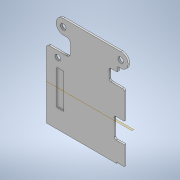
# Autodesk Inventor part: kommutation_board
Saved by Autodesk Inventor 2022 (Build 260153000, 153)
## iProperties
Created: 2024-12-13
Part Number: kommutation_board
Material: Типовые
Document SubType Name: Modeling
Designer: Andrey
Density: 1 g/cm^3
Appearance: По умолчанию
Author: Andrey
Autodesk Inventor part; units mm, degrees
ref_plane "YZ Plane" through (0, 0, 0) normal (1, 0, 0) x (0, 1, 0)
ref_plane "XZ Plane" through (0, 0, 0) normal (0, 1, 0) x (-1, 0, 0)
ref_plane "XY Plane" through (0, 0, 0) normal (0, 0, 1) x (1, 0, 0)
sketch "Эскиз1" plane through (0, 0, 0) normal (0, 0, 1) x (1, 0, 0)
  line L0 (-7.7719, -54) -> (-12.7719, -54) projected
  line L1 (-12.7719, -54) -> (-12.7719, -40.5) projected
  line L2 (-12.7719, -40.5) -> (-7.7719, -40.5) projected
  line L3 (-7.7719, -40.5) -> (-7.7719, -54) projected
  circle A0 centre (-17.7467, 10.9) radius 1.6 projected
  circle A1 centre (-17.7467, -40.1) radius 1.6 projected
  arc A2 (20.7533, -26.4) -> (20.2533, -25.9) centre (20.2533, -26.4) ccw projected
  line L4 (20.2533, -25.9) -> (-21.1, -25.9) projected
  arc A3 (-23.1, -23.9) -> (-21.1, -25.9) centre (-21.1, -23.9) ccw projected
  line L5 (-23.1, -23.9) -> (-23.1, -2.3) projected
  arc A4 (-21.1, -0.3) -> (-23.1, -2.3) centre (-21.1, -2.3) ccw projected
  line L6 (-21.1, -0.3) -> (-13.1, -0.3) projected
  arc A5 (-13.1, -0.3) -> (-11.1, 1.7) centre (-13.1, 1.7) ccw projected
  line L7 (-11.1, 1.7) -> (-11.1, 15.1) projected
  arc A6 (-11.1, 15.1) -> (-13.1, 17.1) centre (-13.1, 15.1) ccw projected
  line L8 (-13.1, 17.1) -> (-15.05, 17.1) projected
  arc A7 (-18.0974, 25.0287) -> (-15.05, 17.1) centre (-15.05, 21.65) ccw projected
  arc A8 (-18.0974, 25.0287) -> (-18.4323, 25.9) centre (-18.4323, 25.4) ccw projected
  line L9 (-25.3018, 25.9) -> (-18.4323, 25.9) projected
  line L10 (-25.3018, 25.9) -> (-25.3018, 22.9) projected
  line L11 (-26.6467, 22.9) -> (-25.3018, 22.9) projected
  line L12 (-26.6467, -42.7) -> (-26.6467, 22.9) projected
  line L13 (-26.6467, -42.7) -> (-18.7719, -42.7) projected
  line L14 (-18.7719, -42.7) -> (-18.7719, -54.2) projected
  line L15 (-18.7719, -54.2) -> (-25.3018, -54.2) projected
  line L16 (-25.3018, -54.2) -> (-25.3018, -55.1) projected
  line L17 (31.7533, -55.1) -> (-25.3018, -55.1) projected
  line L18 (31.7533, -55.1) -> (31.7533, -46.6) projected
  line L19 (31.7533, -46.6) -> (17.9318, -46.6) projected
  spline S0 degree 3 poles (17.3769, -46.1) (17.3769, -46.1597) (17.3919, -46.2298) (17.441, -46.342) (17.485, -46.4032) (17.5795, -46.4922) (17.6478, -46.5345) (17.7766, -46.5847) (17.8606, -46.6) (17.9318, -46.6) knots 0 0 0 0 0.017914 0.017914 0.036753 0.036753 0.056849 0.056849 0.078208 0.078208 0.078208 0.078208 projected
  line L20 (17.3769, -46.1) -> (17.3769, -44.1) projected
  spline S1 degree 3 poles (16.8292, -43.6) (16.8984, -43.6) (16.9801, -43.6153) (17.1065, -43.6649) (17.1743, -43.7071) (17.2685, -43.796) (17.3126, -43.8574) (17.3619, -43.9699) (17.3769, -44.0401) (17.3769, -44.1) knots 0.386783 0.386783 0.386783 0.386783 0.407551 0.407551 0.427519 0.427519 0.446405 0.446405 0.464367 0.464367 0.464367 0.464367 projected
  line L21 (16.8292, -43.6) -> (14.9, -43.6) projected
  line L22 (14.9, -43.6) -> (14.9, -36.8) projected
  line L23 (14.9, -36.8) -> (31.7533, -36.8) projected
  line L24 (31.7533, -36.8) -> (31.7533, -32.1) projected
  line L25 (31.7533, -32.1) -> (20.7533, -32.1) projected
  line L26 (20.7533, -32.1) -> (20.7533, -26.4) projected
  arc A9 (21.8974, 18.2713) -> (22.2323, 17.4) centre (22.2323, 17.9) ccw projected
  line L27 (22.2323, 17.4) -> (31.7533, 17.4) projected
  line L28 (31.7533, 17.4) -> (31.7533, 25.9) projected
  line L29 (22.2323, 25.9) -> (31.7533, 25.9) projected
  arc A10 (22.2323, 25.9) -> (21.8974, 25.0287) centre (22.2323, 25.4) ccw projected
  arc A11 (21.8974, 18.2713) -> (21.8974, 25.0287) centre (18.85, 21.65) ccw projected
  line L30 (21.5533, 2.9) -> (31.7533, 2.9) projected
  line L31 (31.7533, 2.9) -> (31.7533, 7.6) projected
  line L32 (31.7533, 7.6) -> (21.5533, 7.6) projected
  line L33 (7.4642, -8.6) -> (7.4642, -4.1) projected
  line L34 (20.7533, -8.6) -> (7.4642, -8.6) projected
  line L35 (20.7533, 2.9) -> (20.7533, -8.6) projected
  line L36 (21.5533, 2.9) -> (20.7533, 2.9) projected
  line L37 (14.9, 7.6) -> (21.5533, 7.6) projected
  line L38 (14.9, -1.1) -> (14.9, 7.6) projected
  arc A12 (11.9, -4.1) -> (14.9, -1.1) centre (11.9, -1.1) ccw projected
  line L39 (7.4642, -4.1) -> (11.9, -4.1) projected
  line L40 (7.4642, -4.1) -> (11.9, -4.1) projected
  circle A13 centre (-15.05, 21.65) radius 1.5 projected
  line L41 (-18.4323, 25.9) -> (-11.1, 25.9) projected
  arc A14 (-18.0974, 25.0287) -> (-18.4323, 25.9) centre (-18.4323, 25.4) ccw projected
  arc A15 (-18.0974, 25.0287) -> (-15.05, 17.1) centre (-15.05, 21.65) ccw projected
  line L42 (-13.1, 17.1) -> (-15.05, 17.1) projected
  arc A16 (-11.1, 15.1) -> (-13.1, 17.1) centre (-13.1, 15.1) ccw projected
  line L43 (-11.1, 25.9) -> (-11.1, 15.1) projected
  line L44 (14.9, 25.9) -> (22.2323, 25.9) projected
  line L45 (14.9, 14.4) -> (14.9, 25.9) projected
  line L46 (16.4121, 14.4) -> (14.9, 14.4) projected
  spline S2 degree 3 poles (16.9309, 14.9) (16.9309, 14.839) (16.9162, 14.7674) (16.8681, 14.654) (16.8258, 14.5925) (16.7358, 14.5046) (16.6718, 14.463) (16.5529, 14.4148) (16.4768, 14.4) (16.4121, 14.4) knots 0.150725 0.150725 0.150725 0.150725 0.169014 0.169014 0.187674 0.187674 0.206759 0.206759 0.226155 0.226155 0.226155 0.226155 projected
  line L47 (16.9309, 16.9) -> (16.9309, 14.9) projected
  spline S3 degree 3 poles (17.4522, 17.4) (17.3868, 17.4) (17.3098, 17.3852) (17.1901, 17.3368) (17.1259, 17.2952) (17.0358, 17.2072) (16.9935, 17.1458) (16.9455, 17.0325) (16.9309, 16.9609) (16.9309, 16.9) knots -0.075652 -0.075652 -0.075652 -0.075652 -0.056047 -0.056047 -0.036914 -0.036914 -0.018271 -0.018271 0 0 0 0 projected
  line L48 (22.2323, 17.4) -> (17.4522, 17.4) projected
  arc A17 (21.8974, 18.2713) -> (22.2323, 17.4) centre (22.2323, 17.9) ccw projected
  arc A18 (21.8974, 18.2713) -> (21.8974, 25.0287) centre (18.85, 21.65) ccw projected
  arc A19 (22.2323, 25.9) -> (21.8974, 25.0287) centre (22.2323, 25.4) ccw projected
  circle A20 centre (18.85, 21.65) radius 1.5 projected
  circle A21 centre (18.85, 21.65) radius 4.25
  circle A22 centre (-15.05, 21.65) radius 4.25
  line L49 (18.85, 25.9) -> (-15.05, 25.9)
  circle A23 centre (18.85, 21.65) radius 1.6
  circle A24 centre (-15.05, 21.65) radius 1.6
  line L50 (14.9, 7.6) -> (12.9, 7.6)
  line L51 (11.9, 8.6) -> (11.9, 13.4)
  line L52 (12.9, 14.4) -> (14.9, 14.4)
  line L53 (14.9, 14.4) -> (14.9, 7.6)
  line L54 (20.7533, -25.6) -> (-21.1, -25.6)
  arc A25 (-22.8, -23.9) -> (-21.1, -25.6) centre (-21.1, -23.9) ccw
  line L55 (-22.8, -23.9) -> (-22.8, -2.3)
  line L56 (-21.1, -0.6) -> (-13.1, -0.6)
  arc A26 (-13.1, -0.6) -> (-10.8, 1.7) centre (-13.1, 1.7) ccw
  arc A27 (-21.1, -0.6) -> (-22.8, -2.3) centre (-21.1, -2.3) ccw
  line L57 (-10.8, 1.7) -> (-10.8, 15.1)
  arc A28 (-10.8, 15.1) -> (-13.1, 17.4) centre (-13.1, 15.1) ccw
  line L58 (-13.1, 17.4) -> (-15.05, 17.4)
  arc A29 (21.0533, 3.4) -> (21.5533, 2.9) centre (21.5533, 3.4) ccw projected
  arc A30 (21.5533, 7.6) -> (21.0533, 7.1) centre (21.5533, 7.1) ccw projected
  line L59 (21.0533, 7.1) -> (21.0533, 3.4) projected
  arc A31 (21.0533, 3.4) -> (21.5533, 2.9) centre (21.5533, 3.4) ccw projected
  line L60 (21.0533, 7.1) -> (21.0533, 3.4) projected
  arc A32 (21.5533, 7.6) -> (21.0533, 7.1) centre (21.5533, 7.1) ccw projected
  line L61 (20.7533, 2.9) -> (20.7533, 6.6)
  line L62 (19.7533, 7.6) -> (14.9, 7.6)
  arc A33 (20.7533, 6.6) -> (19.7533, 7.6) centre (19.7533, 6.6) ccw
  arc A34 (11.9, 8.6) -> (12.9, 7.6) centre (12.9, 8.6) ccw
  arc A35 (12.9, 14.4) -> (11.9, 13.4) centre (12.9, 13.4) ccw
  line L63 (20.7533, -25.6) -> (20.7533, -20.6)
  line L64 (20.7533, -20.6) -> (15.9, -20.6)
  line L65 (20.7533, -8.6) -> (7.4642, -8.6) projected
  line L66 (20.7533, 2.9) -> (20.7533, -8.6) projected
  line L67 (21.5533, 2.9) -> (20.7533, 2.9) projected
  arc A36 (21.0533, 3.4) -> (21.5533, 2.9) centre (21.5533, 3.4) ccw projected
  line L68 (21.0533, 7.1) -> (21.0533, 3.4) projected
  arc A37 (21.5533, 7.6) -> (21.0533, 7.1) centre (21.5533, 7.1) ccw projected
  line L69 (14.9, 7.6) -> (21.5533, 7.6) projected
  line L70 (14.9, -1.1) -> (14.9, 7.6) projected
  arc A38 (11.9, -4.1) -> (14.9, -1.1) centre (11.9, -1.1) ccw projected
  line L71 (7.4642, -8.6) -> (7.4642, -4.1) projected
  arc A39 (14.9, -19.6) -> (15.9, -20.6) centre (15.9, -19.6) ccw projected
  line L72 (14.9, -19.6) -> (14.9, -9.6) projected
  arc A40 (15.9, -8.6) -> (14.9, -9.6) centre (15.9, -9.6) ccw projected
  line L73 (-7.7719, -54) -> (-12.7719, -54) projected
  line L74 (-12.7719, -54) -> (-12.7719, -40.5) projected
  line L75 (-12.7719, -40.5) -> (-7.7719, -40.5) projected
  line L76 (-7.7719, -40.5) -> (-7.7719, -54) projected
  circle A41 centre (-17.7467, 10.9) radius 1.6 projected
  circle A42 centre (-17.7467, -40.1) radius 1.6 projected
  arc A43 (20.7533, -26.4) -> (20.2533, -25.9) centre (20.2533, -26.4) ccw projected
  line L77 (20.2533, -25.9) -> (-21.1, -25.9) projected
  arc A44 (-23.1, -23.9) -> (-21.1, -25.9) centre (-21.1, -23.9) ccw projected
  line L78 (-23.1, -23.9) -> (-23.1, 4.7) projected
  arc A45 (-21.1, 6.7) -> (-23.1, 4.7) centre (-21.1, 4.7) ccw projected
  line L79 (-21.1, 6.7) -> (-13.1, 6.7) projected
  arc A46 (-13.1, 6.7) -> (-11.1, 8.7) centre (-13.1, 8.7) ccw projected
  line L80 (-11.1, 8.7) -> (-11.1, 15.1) projected
  arc A47 (-11.1, 15.1) -> (-13.1, 17.1) centre (-13.1, 15.1) ccw projected
  line L81 (-13.1, 17.1) -> (-15.05, 17.1) projected
  arc A48 (-18.0974, 25.0287) -> (-15.05, 17.1) centre (-15.05, 21.65) ccw projected
  arc A49 (-18.0974, 25.0287) -> (-18.4323, 25.9) centre (-18.4323, 25.4) ccw projected
  line L82 (-25.3018, 25.9) -> (-18.4323, 25.9) projected
  line L83 (-25.3018, 25.9) -> (-25.3018, 22.9) projected
  line L84 (-26.6467, 22.9) -> (-25.3018, 22.9) projected
  line L85 (-26.6467, -42.7) -> (-26.6467, 22.9) projected
  line L86 (-26.6467, -42.7) -> (-18.7719, -42.7) projected
  line L87 (-18.7719, -42.7) -> (-18.7719, -54.2) projected
  line L88 (-18.7719, -54.2) -> (-25.3018, -54.2) projected
  line L89 (-25.3018, -54.2) -> (-25.3018, -55.1) projected
  line L90 (31.7533, -55.1) -> (-25.3018, -55.1) projected
  line L91 (31.7533, -55.1) -> (31.7533, -46.6) projected
  line L92 (31.7533, -46.6) -> (17.9318, -46.6) projected
  spline S4 degree 3 poles (17.3769, -46.1) (17.3769, -46.1597) (17.3919, -46.2298) (17.441, -46.342) (17.485, -46.4032) (17.5795, -46.4922) (17.6478, -46.5345) (17.7766, -46.5847) (17.8606, -46.6) (17.9318, -46.6) knots 0 0 0 0 0.017914 0.017914 0.036753 0.036753 0.056849 0.056849 0.078208 0.078208 0.078208 0.078208 projected
  line L93 (17.3769, -46.1) -> (17.3769, -44.1) projected
  spline S5 degree 3 poles (16.8292, -43.6) (16.8984, -43.6) (16.9801, -43.6153) (17.1065, -43.6649) (17.1743, -43.7071) (17.2685, -43.796) (17.3126, -43.8574) (17.3619, -43.9699) (17.3769, -44.0401) (17.3769, -44.1) knots 0.386783 0.386783 0.386783 0.386783 0.407551 0.407551 0.427519 0.427519 0.446405 0.446405 0.464367 0.464367 0.464367 0.464367 projected
  line L94 (16.8292, -43.6) -> (14.9, -43.6) projected
  line L95 (14.9, -43.6) -> (14.9, -36.8) projected
  line L96 (14.9, -36.8) -> (31.7533, -36.8) projected
  line L97 (31.7533, -36.8) -> (31.7533, -32.1) projected
  line L98 (31.7533, -32.1) -> (20.7533, -32.1) projected
  line L99 (20.7533, -32.1) -> (20.7533, -26.4) projected
  line L100 (-10.8, 15.1) -> (-10.8, 8.7)
  arc A50 (-13.1, 6.4) -> (-10.8, 8.7) centre (-13.1, 8.7) ccw
  line L101 (-13.1, 6.4) -> (-21.1, 6.4)
  arc A51 (-21.1, 6.4) -> (-22.8, 4.7) centre (-21.1, 4.7) ccw
  line L102 (-22.8, 4.7) -> (-22.8, -23.9)
  line L103 (-7.7719, -54) -> (-12.7719, -54) projected
  line L104 (-12.7719, -54) -> (-12.7719, -40.5) projected
  line L105 (-12.7719, -40.5) -> (-7.7719, -40.5) projected
  line L106 (-7.7719, -40.5) -> (-7.7719, -54) projected
  circle A52 centre (-17.7467, 10.9) radius 1.6 projected
  circle A53 centre (-17.7467, -40.1) radius 1.6 projected
  arc A54 (20.7533, -29.4) -> (20.2533, -28.9) centre (20.2533, -29.4) ccw projected
  line L107 (20.2533, -28.9) -> (-21.1, -28.9) projected
  arc A55 (-23.1, -26.9) -> (-21.1, -28.9) centre (-21.1, -26.9) ccw projected
  line L108 (-23.1, -26.9) -> (-23.1, 4.7) projected
  arc A56 (-21.1, 6.7) -> (-23.1, 4.7) centre (-21.1, 4.7) ccw projected
  line L109 (-21.1, 6.7) -> (-13.1, 6.7) projected
  arc A57 (-13.1, 6.7) -> (-11.1, 8.7) centre (-13.1, 8.7) ccw projected
  line L110 (-11.1, 8.7) -> (-11.1, 15.1) projected
  arc A58 (-11.1, 15.1) -> (-13.1, 17.1) centre (-13.1, 15.1) ccw projected
  line L111 (-13.1, 17.1) -> (-15.05, 17.1) projected
  arc A59 (-18.0974, 25.0287) -> (-15.05, 17.1) centre (-15.05, 21.65) ccw projected
  arc A60 (-18.0974, 25.0287) -> (-18.4323, 25.9) centre (-18.4323, 25.4) ccw projected
  line L112 (-25.3018, 25.9) -> (-18.4323, 25.9) projected
  line L113 (-25.3018, 25.9) -> (-25.3018, 22.9) projected
  line L114 (-26.6467, 22.9) -> (-25.3018, 22.9) projected
  line L115 (-26.6467, -42.7) -> (-26.6467, 22.9) projected
  line L116 (-26.6467, -42.7) -> (-18.7719, -42.7) projected
  line L117 (-18.7719, -42.7) -> (-18.7719, -54.2) projected
  line L118 (-18.7719, -54.2) -> (-25.3018, -54.2) projected
  line L119 (-25.3018, -54.2) -> (-25.3018, -55.1) projected
  line L120 (31.7533, -55.1) -> (-25.3018, -55.1) projected
  line L121 (31.7533, -55.1) -> (31.7533, -46.6) projected
  line L122 (31.7533, -46.6) -> (17.9318, -46.6) projected
  spline S6 degree 3 poles (17.3769, -46.1) (17.3769, -46.1597) (17.3919, -46.2298) (17.441, -46.342) (17.485, -46.4032) (17.5795, -46.4922) (17.6478, -46.5345) (17.7766, -46.5847) (17.8606, -46.6) (17.9318, -46.6) knots 0 0 0 0 0.017914 0.017914 0.036753 0.036753 0.056849 0.056849 0.078208 0.078208 0.078208 0.078208 projected
  line L123 (17.3769, -46.1) -> (17.3769, -44.1) projected
  spline S7 degree 3 poles (16.8292, -43.6) (16.8984, -43.6) (16.9801, -43.6153) (17.1065, -43.6649) (17.1743, -43.7071) (17.2685, -43.796) (17.3126, -43.8574) (17.3619, -43.9699) (17.3769, -44.0401) (17.3769, -44.1) knots 0.386783 0.386783 0.386783 0.386783 0.407551 0.407551 0.427519 0.427519 0.446405 0.446405 0.464367 0.464367 0.464367 0.464367 projected
  line L124 (16.8292, -43.6) -> (14.9, -43.6) projected
  line L125 (14.9, -43.6) -> (14.9, -36.8) projected
  line L126 (14.9, -36.8) -> (31.7533, -36.8) projected
  line L127 (31.7533, -36.8) -> (31.7533, -32.1) projected
  line L128 (31.7533, -32.1) -> (20.7533, -32.1) projected
  line L129 (20.7533, -32.1) -> (20.7533, -29.4) projected
  line L130 (-22.8, 4.7) -> (-22.8, -26.9)
  arc A61 (-22.8, -26.9) -> (-21.1, -28.6) centre (-21.1, -26.9) ccw
  line L131 (-21.1, -28.6) -> (20.7533, -28.6)
  line L132 (21.0533, -29.4) -> (21.0533, -32.1)
  line L133 (20.7533, -28.6) -> (20.7533, -25.6)
  arc A62 (-23.3497, 8.2) -> (-25.3497, 6.2) centre (-23.3497, 6.2) ccw
  line L134 (-23.3497, 8.2) -> (-13.1, 8.2)
  arc A63 (-13.1, 8.2) -> (-11.1, 10.2) centre (-13.1, 10.2) ccw
  line L135 (-25.3497, 0.9) -> (-25.3497, 6.2)
  line L136 (-25.3499, -32.7) -> (-25.3499, 0.9)
  line L137 (16.4642, -32.7) -> (-25.3499, -32.7)
  line L138 (31.7533, -32.1) -> (16.4642, -32.1)
  line L139 (16.4642, -32.1) -> (16.4642, -32.7)
  line L140 (31.7533, -31.8) -> (16.1642, -31.8)
  line L141 (16.1642, -31.8) -> (16.1642, -32.4)
  line L142 (16.1642, -32.4) -> (-25.0499, -32.4)
  line L143 (-25.0499, -32.4) -> (-25.0499, 0.9)
  line L144 (-25.0497, 0.9) -> (-25.0497, 6.2)
  arc A64 (-23.3497, 7.9) -> (-25.0497, 6.2) centre (-23.3497, 6.2) ccw
  line L145 (-23.3497, 7.9) -> (-13.1, 7.9)
  arc A65 (-13.1, 7.9) -> (-10.8, 10.2) centre (-13.1, 10.2) ccw
  line L146 (-10.8, 10.2) -> (-10.8, 15.1)
  line L147 (20.7533, -28.6) -> (20.7533, -31.8)
  line L148 (20.7533, -28.6) -> (-21.1, -28.6)
  line L149 (-25.0499, -32.4) -> (16.1642, -32.4)
  line L150 (16.1642, -31.8) -> (16.1642, -32.4)
  line L151 (16.1642, -31.8) -> (20.7533, -31.8)
  line L152 (-25.0497, 6.2) -> (-25.0499, -32.4)
  line L153 (-10.8, 10.2) -> (-10.8, 1.7)
  point P0 (0, 0)
  point P1 (20.7533, 3.4)
  point P2 (20.7533, 7.1)
  point P3 (7.4642, -25.9)
  point P4 (-3.6642, -25.9)
  point P5 (11.9, 14.4)
  point P6 (20.7533, 7.6)
  point P7 (18.85, 17.4)
  point P8 (-22.8, -2.3)
  point P9 (-21.1, -25.6)
  point P10 (-11.1, 16.2358)
  point P11 (-22.8, -2.3)
  point P12 (20.7533, -26.4)
  point P13 (-11.1, 9.0642)
  point P14 (-22.8, -1.2464)
  point P15 (-22.8, -2.3)
  dimension "d0" = 3.2
  dimension "d1" = 3.2
  dimension "d2" = 3
  dimension "d3" = 0.3
  dimension "d4" = 0.3
  dimension "d5" = 0.3
  dimension "d6" = 0.3
  dimension "d7" = 0.3
  dimension "d8" = 0.3
  dimension "d9" = 0.3
  dimension "d10" = 0.3
  dimension "d11" = 0.3
  dimension "d12" = 1
  dimension "d13" = 1
  dimension "d20" = 0.3
  dimension "d22" = 0.3
  dimension "d26" = 0.3
  dimension "d27" = 0.3
  constraints: 82 end point, 28 point on circle, 16 centre point, 10 point on line, 10 tangent, 8 parallel, 6 horizontal, 5 perpendicular, 4 coincident, 4 vertical, 3 collinear, 1 equal radius, 32 other
  measures "d0" diameter of A23
  measures "d1" diameter of A24
  measures "d2" distance of point (11.9, 14.4) L52.end
  measures "d3" distance between parallel lines of L4 L54
  measures "d4" radial gap between concentric circles of A3 A25
  measures "d5" distance between parallel lines of L5 L55
  measures "d6" distance between parallel lines of L6 L56
  measures "d7" radial gap between concentric circles of A5 A26
  measures "d8" radial gap between concentric circles of A4 A27
  measures "d9" distance between parallel lines of L7 L57
  measures "d10" radial gap between concentric circles of A6 A28
  measures "d11" distance between parallel lines of L8 L58
  measures "d12" radius of A33
  measures "d13" radius of A34
  measures "d20" radial gap between concentric circles of A46 A50
  measures "d22" distance between parallel lines of L107 L131
  measures "d26" distance between parallel lines of L138 L140
  measures "d27" radial gap between concentric circles of A62 A64
extrude "Выдавливание1" add sketch "Эскиз1" along normal blind 1 contours L26 L131 A61 L130 A3 L4 A2 | A2 L4 A3 L130 A25 L54 L133 | L26 A54 L107 A55 L108 A3 L130 A61 L131 | L54 A25 L55 A27 L56 A26 L57 A28 L43 A22 L49 L45 A21 L52 A35 L51 A34 L50 L38 A12 L39 L33 L34 A40 L72 A39 L64 L63 | L26 L140 L141 L142 L143 L144 A64 L145 A65 L7 A46 L79 A45 L78 L5 L108 A55 L107 A54 | A3 L5 A4 L102 L55 L130 | L102 A4 L6 A5 L7 A50 L57 A26 L56 A27 | L78 A45 L79 A46 L7 A50 L101 A51 L102 A4 | L102 A51 L101 A50 L7 A5 L6 A4 | L34 L33 L39 A12 L38 L37 A33 L61 L35 | A50 L7 A65 L57 | A28 L58 A22 L43 | A22 L43 | L43 A22 | L45 A21 L48 S3 L47 S2 L46 | A22 L41 L43 | A21 L45 | L45 A21 | L45 L44 A21
sketch "Эскиз2" plane through (0, 0, 1) normal (0, 0, 1) x (1, 0, 0)
  circle A0 centre (-18.2249, 4.4) radius 2.1
  circle A1 centre (-18.2249, 4.4) radius 1.6
  point P0 (0, 0)
  dimension "d29" = 3.2
  constraints: 2 centre point, 1 coincident, 2 other
  measures "d29" diameter of A1
extrude "Выдавливание2" cut sketch "Эскиз2" against normal blind 1 contours A1
ref_plane "РабПлоскость1" through (-21.1, -11.1, 0) normal (0, 1, 0) x (1, 0, 0)
sketch "Эскиз3" plane through (0, 0, 1) normal (0, 0, 1) x (1, 0, 0)
  line L0 (-17.15, -1.45) -> (-18.45, -1.45) projected
  line L1 (-17.15, -2.75) -> (-17.15, -1.45) projected
  line L2 (-18.45, -2.75) -> (-17.15, -2.75) projected
  line L3 (-18.45, -1.45) -> (-18.45, -2.75) projected
  line L4 (-17.15, -3.45) -> (-18.45, -3.45) projected
  line L5 (-17.15, -4.75) -> (-17.15, -3.45) projected
  line L6 (-18.45, -4.75) -> (-17.15, -4.75) projected
  line L7 (-18.45, -3.45) -> (-18.45, -4.75) projected
  line L8 (-18.4122, -10.7426) -> (-17.1122, -10.7426) projected
  line L9 (-18.4122, -9.4426) -> (-18.4122, -10.7426) projected
  line L10 (-17.1122, -9.4426) -> (-18.4122, -9.4426) projected
  line L11 (-17.1122, -10.7426) -> (-17.1122, -9.4426) projected
  line L12 (-17.15, -11.45) -> (-18.45, -11.45) projected
  line L13 (-17.15, -12.75) -> (-17.15, -11.45) projected
  line L14 (-18.45, -12.75) -> (-17.15, -12.75) projected
  line L15 (-18.45, -11.45) -> (-18.45, -12.75) projected
  line L16 (-16.45, -18.75) -> (-15.15, -18.75) projected
  line L17 (-16.45, -17.45) -> (-16.45, -18.75) projected
  line L18 (-15.15, -17.45) -> (-16.45, -17.45) projected
  line L19 (-15.15, -18.75) -> (-15.15, -17.45) projected
  line L20 (-16.45, -16.75) -> (-15.15, -16.75) projected
  line L21 (-16.45, -15.45) -> (-16.45, -16.75) projected
  line L22 (-15.15, -15.45) -> (-16.45, -15.45) projected
  line L23 (-15.15, -16.75) -> (-15.15, -15.45) projected
  line L24 (-18.45, -8.75) -> (-17.15, -8.75) projected
  line L25 (-18.45, -7.45) -> (-18.45, -8.75) projected
  line L26 (-17.15, -7.45) -> (-18.45, -7.45) projected
  line L27 (-17.15, -8.75) -> (-17.15, -7.45) projected
  line L28 (-15.15, -11.45) -> (-16.45, -11.45) projected
  line L29 (-15.15, -12.75) -> (-15.15, -11.45) projected
  line L30 (-16.45, -12.75) -> (-15.15, -12.75) projected
  line L31 (-16.45, -11.45) -> (-16.45, -12.75) projected
  line L32 (-16.45, -20.75) -> (-15.15, -20.75) projected
  line L33 (-16.45, -19.45) -> (-16.45, -20.75) projected
  line L34 (-15.15, -19.45) -> (-16.45, -19.45) projected
  line L35 (-15.15, -20.75) -> (-15.15, -19.45) projected
  line L36 (-15.15, -5.45) -> (-16.45, -5.45) projected
  line L37 (-15.15, -6.75) -> (-15.15, -5.45) projected
  line L38 (-16.45, -6.75) -> (-15.15, -6.75) projected
  line L39 (-16.45, -5.45) -> (-16.45, -6.75) projected
  line L40 (-18.8, -0.9) -> (-18.8, -21.3) projected
  line L41 (-18.8, -21.3) -> (-14.8, -21.3) projected
  line L42 (-14.8, -21.3) -> (-14.8, -0.9) projected
  line L43 (-14.8, -0.9) -> (-18.8, -0.9) projected
  line L44 (-18.45, -5.45) -> (-18.45, -6.75) projected
  line L45 (-17.15, -5.45) -> (-18.45, -5.45) projected
  line L46 (-17.15, -6.75) -> (-17.15, -5.45) projected
  line L47 (-18.45, -6.75) -> (-17.15, -6.75) projected
  line L48 (-17.15, -19.45) -> (-18.45, -19.45) projected
  line L49 (-17.15, -20.75) -> (-17.15, -19.45) projected
  line L50 (-18.45, -20.75) -> (-17.15, -20.75) projected
  line L51 (-18.45, -19.45) -> (-18.45, -20.75) projected
  line L52 (-16.45, -14.75) -> (-15.15, -14.75) projected
  line L53 (-16.45, -13.45) -> (-16.45, -14.75) projected
  line L54 (-15.15, -13.45) -> (-16.45, -13.45) projected
  line L55 (-15.15, -14.75) -> (-15.15, -13.45) projected
  line L56 (-17.15, -13.45) -> (-18.45, -13.45) projected
  line L57 (-17.15, -14.75) -> (-17.15, -13.45) projected
  line L58 (-18.45, -14.75) -> (-17.15, -14.75) projected
  line L59 (-18.45, -13.45) -> (-18.45, -14.75) projected
  line L60 (-17.15, -17.45) -> (-18.45, -17.45) projected
  line L61 (-17.15, -18.75) -> (-17.15, -17.45) projected
  line L62 (-18.45, -18.75) -> (-17.15, -18.75) projected
  line L63 (-18.45, -17.45) -> (-18.45, -18.75) projected
  line L64 (-17.15, -15.45) -> (-18.45, -15.45) projected
  line L65 (-17.15, -16.75) -> (-17.15, -15.45) projected
  line L66 (-18.45, -16.75) -> (-17.15, -16.75) projected
  line L67 (-18.45, -15.45) -> (-18.45, -16.75) projected
  line L68 (-15.15, -9.45) -> (-16.45, -9.45) projected
  line L69 (-15.15, -10.75) -> (-15.15, -9.45) projected
  line L70 (-16.45, -10.75) -> (-15.15, -10.75) projected
  line L71 (-16.45, -9.45) -> (-16.45, -10.75) projected
  line L72 (-15.15, -7.45) -> (-16.45, -7.45) projected
  line L73 (-15.15, -8.75) -> (-15.15, -7.45) projected
  line L74 (-16.45, -8.75) -> (-15.15, -8.75) projected
  line L75 (-16.45, -7.45) -> (-16.45, -8.75) projected
  line L76 (-16.45, -4.75) -> (-15.15, -4.75) projected
  line L77 (-16.45, -3.45) -> (-16.45, -4.75) projected
  line L78 (-15.15, -3.45) -> (-16.45, -3.45) projected
  line L79 (-15.15, -4.75) -> (-15.15, -3.45) projected
  line L80 (-15.15, -2.75) -> (-15.15, -1.45) projected
  line L81 (-16.45, -2.75) -> (-15.15, -2.75) projected
  line L82 (-16.45, -1.45) -> (-16.45, -2.75) projected
  line L83 (-15.15, -1.45) -> (-16.45, -1.45) projected
  point P0 (0, 0)
extrude "Выдавливание3" cut sketch "Эскиз3" against normal blind 0.5 contours L1 L2 L3 L0 | L5 L6 L7 L4 | L9 L10 L11 L8 | L13 L14 L15 L12 | L17 L18 L19 L16 | L21 L22 L23 L20 | L25 L26 L27 L24 | L29 L30 L31 L28 | L33 L34 L35 L32 | L37 L38 L39 L36 | L43 L42 L41 L40 | L45 L46 L47 L44 | L49 L50 L51 L48 | L53 L54 L55 L52 | L57 L58 L59 L56 | L61 L62 L63 L60 | L65 L66 L67 L64 | L69 L70 L71 L68 | L73 L74 L75 L72 | L77 L78 L79 L76 | L81 L82 L83 L80
